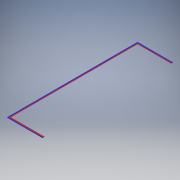
# Autodesk Inventor part: Trim_Blue
Saved by Autodesk Inventor 2017.1 (Build 211199000, 199)
## iProperties
Created: 2017-01-05
Part Number: Trim_Blue
Material: Generic
Document SubType Name: Modeling
Designer: PhillipD
Density: 1 g/cm^3
Appearance: Blue - Wall Paint - Glossy
Author: PhillipD
Autodesk Inventor part; units mm, degrees
ref_plane "YZ Plane" through (0, 0, 0) normal (1, 0, 0) x (0, 1, 0)
ref_plane "XZ Plane" through (0, 0, 0) normal (0, 1, 0) x (-1, 0, 0)
ref_plane "XY Plane" through (0, 0, 0) normal (0, 0, 1) x (1, 0, 0)
sketch "Sketch1" plane through (0, 0, 0) normal (0, 1, 0) x (-1, 0, 0)
  line L0 (0, 0) -> (1922.78, 0)
  line L1 (1922.78, 0) -> (1922.78, -7045.96)
  line L2 (1922.78, -7045.96) -> (0, -7045.96)
  line L3 (0, -6995.16) -> (1871.98, -6995.16)
  line L4 (1871.98, -6995.16) -> (1871.98, -50.8)
  line L5 (1871.98, -50.8) -> (0, -50.8)
  line L6 (0, 0) -> (0, -50.8)
  line L7 (0, -6995.16) -> (0, -7045.96)
  line L8 (1821.18, -6944.36) -> (0, -6944.36)
  line L9 (1821.18, -6944.36) -> (1821.18, -119.7177)
  line L10 (0, -6944.36) -> (0, -6995.16)
  line L11 (1821.18, -119.7177) -> (0, -119.7177)
  line L12 (0, -50.8) -> (0, -119.7177)
  dimension "d0" = 1922.78
  dimension "d1" = 7045.96
  dimension "d2" = 1922.78
  dimension "d3" = 50.8
  dimension "d6" = 50.8
  dimension "d7" = 50.8
  constraints: 26 end point, 4 perpendicular, 4 vertical, 3 horizontal, 1 collinear, 2 other
  measures "d0" distance of L0.start L0.end
  measures "d1" distance of L0.end L1.end
  measures "d2" distance of L1.end L2.end
  measures "d3" distance between parallel lines of L1 L4
  measures "d6" distance between parallel lines of L8 L3
  measures "d7" distance between parallel lines of L4 L9
extrude "Extrusion1" add sketch "Sketch1" along normal blind 3.175 contours L0 L1 L2 L7 L3 L4 L5 L6
extrude "Extrusion2" add sketch "Sketch1" along normal blind 3.175 separate body contours L5 L4 L3 L10 L8 L9 L11 L12
equation "\"d0\" = d2"
body "Solid1"
body "Solid2"
